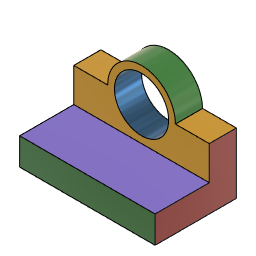
Ex 2 v2 (Autodesk Fusion 360 design; units mm, degrees)
Autodesk Fusion 360 part; units mm, degrees
sketch "Sketch1" plane through (0, 0, 0) normal (0, 0, 1) x (1, 0, 0)
  line L0 (50, 30) -> (-50, 30)
  line L1 (-50, 30) -> (-50, -30)
  line L2 (-50, -30) -> (50, -30)
  line L3 (50, -30) -> (50, 30)
  line L4 (50, 30) -> (-50, -30) construction
  line L5 (-50, 30) -> (50, -30) construction
  line L6 (-50, 30) -> (-25, 30)
  line L7 (-25, 30) -> (-25, 10)
  line L8 (-25, 10) -> (-50, 10)
  line L9 (-50, 10) -> (-50, 30)
  line L10 (-25, 30) -> (25, 30)
  line L11 (25, 30) -> (25, 10)
  line L12 (25, 10) -> (-25, 10)
  line L13 (-25, 10) -> (-25, 30)
  line L14 (25, 30) -> (50, 30)
  line L15 (50, 30) -> (50, 10)
  line L16 (50, 10) -> (25, 10)
  line L17 (25, 10) -> (25, 30)
  dimension "d1" = 100
  dimension "d2" = 60
  dimension "d3" = 25
  dimension "d4" = 50
  dimension "d5" = 20
  constraint horizontal L0
  constraint perpendicular L0 L1
  constraint parallel L0 L2
  constraint parallel L1 L3
  constraint coincident L4 origin
  constraint coincident L5 origin
  constraint horizontal L6
  constraint vertical L7
  constraint horizontal L8
  constraint vertical L9
  constraint horizontal L10
  constraint vertical L11
  constraint horizontal L12
  constraint vertical L13
  constraint horizontal L14
  constraint vertical L15
  constraint horizontal L16
  constraint vertical L17
  constraint coincident L3 L15.end
  measures "d1" distance of L1.end L2.end
  measures "d2" distance of L0.end L1.end
  measures "d3" distance of L0.end L6.end
  measures "d4" distance of L6.end L10.end
  measures "d5" distance of L6.end L7.end
extrude "Extrude1" add sketch "Sketch1" along normal blind 20 contours L1 L2 L3 L8 L12 L16
extrude "Extrude2" add sketch "Sketch1" along normal blind 45 contours L0 L3 L11 L14 L15 L16 L17 | L0 L7 L10 L11 L12 L13 L17 | L0 L1 L6 L7 L8 L9 L13
sketch "Sketch2" plane through (0, 0, 0) normal (0, 1, 0) x (1, 0, 0)
sketch "Sketch3" plane through (0, 10, 0) normal (0, -1, 0) x (1, 0, 0)
  line L0 (-50, 20) -> (50, 20)
  line L1 (50, 20) -> (50, 45)
  line L2 (-50, 45) -> (-50, 20)
  circle A0 centre (0, 45) radius 20
  arc A1 (25, 45) -> (-25, 45) centre (0, 45) ccw
  line L3 (-25, 45) -> (-20, 45)
  line L4 (20, 45) -> (25, 45)
  dimension "d10" = 40
  constraint concentric A0 A1
  constraint coincident A0 L3.end
  constraint horizontal L3
  constraint coincident A0 L4.start
  constraint parallel L3 L4
  measures "d10" diameter of A0
hole "Hole1" at (0, 10, 45) direction (0, 1, 0) diameter 40 depth 40 tip angle 118
extrude "Extrude3" add sketch "Sketch3" against normal blind 20 contours A0 A1 L3 L4
sketch "Sketch4" plane through (50, 0, 0) normal (1, 0, 0) x (0, 1, 0)
  line L0 (-30, 0) -> (30, 0)
  line L1 (30, 0) -> (30, 45)
  line L2 (30, 45) -> (10, 45)
  line L3 (10, 45) -> (10, 20)
  line L4 (10, 20) -> (-30, 20)
  line L5 (-30, 20) -> (-30, 0)
